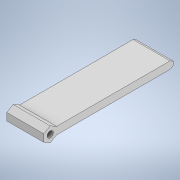
# Autodesk Inventor part: HexFlipper
Saved by Autodesk Inventor 2020 (Build 240168000, 168)
## iProperties
Created: 2023-12-22
Part Number: HexFlipper
Material: Generic
Document SubType Name: Modeling
Designer: smz3rm
Density: 1 g/cm^3
Appearance: Default
Author: smz3rm
Autodesk Inventor part; units mm, degrees
ref_plane "YZ Plane" through (0, 0, 0) normal (1, 0, 0) x (0, 1, 0)
ref_plane "XZ Plane" through (0, 0, 0) normal (0, 1, 0) x (-1, 0, 0)
ref_plane "XY Plane" through (0, 0, 0) normal (0, 0, 1) x (1, 0, 0)
sketch "Sketch1" plane through (0, 0, 0) normal (1, 0, 0) x (0, 1, 0)
  line L0 (2, 35) -> (-2, 35)
  line L1 (-2, 35) -> (-2, -35)
  line L2 (-2, -35) -> (2, -35)
  line L3 (2, -35) -> (2, 35)
  line L4 (2, 35) -> (-2, -35) construction
  line L5 (-2, 35) -> (2, -35) construction
  line L6 (-1, -35) -> (-2, -33.2679)
  line L7 (-2, -33.2679) -> (-1, -31.5359)
  line L8 (-1, -31.5359) -> (1, -31.5359)
  line L9 (1, -31.5359) -> (2, -33.2679)
  line L10 (2, -33.2679) -> (1, -35)
  line L11 (1, -35) -> (-1, -35)
  line L12 (4, 31.5359) -> (2, 28.0718)
  line L13 (2, 28.0718) -> (-2, 28.0718)
  line L14 (-2, 28.0718) -> (-4, 31.5359)
  line L15 (-4, 31.5359) -> (-2, 35)
  line L16 (-2, 35) -> (2, 35)
  line L17 (2, 35) -> (4, 31.5359)
  circle A0 centre (0, 31.5359) radius 1.65
  point P0 (0, 0)
  point P1 (0, -33.2679)
  dimension "d0" = 4
  dimension "d1" = 70
  dimension "d2" = 3.3
  constraints: 36 end point, 4 point on line, 2 midpoint, 2 parallel, 1 centre point, 1 coincident, 1 horizontal, 1 perpendicular, 26 other
  measures "d0" distance of L2.end L1.end
  measures "d1" distance of L1.end L0.end
  measures "d2" diameter of A0
extrude "Extrusion1" add sketch "Sketch1" along normal blind 20 contours L3 L13 L1 L0 | L17 L12 L3 | L1 L14 L15 | L3 L9 L8 L7 L1 L13 | L10 L2 L6 L7 L8 L9
ref_plane "Work Plane1" through (0, 2, 28.0718) normal (0, 0, -1) x (1, 0, 0)
sketch "Sketch2" plane through (0, -1, -35) normal (0, 0, -1) x (-1, 0, 0)
  line L0 (0, 2) -> (-20, 2) projected
  line L1 (0, 0) -> (-20, 0) projected
  line L2 (-10, 2) -> (-10, 0)
  circle A0 centre (-10, 1) radius 1
  point P0 (0, 1)
  dimension "d5" = 2
  constraints: 3 midpoint, 2 end point, 1 centre point, 1 vertical
  measures "d5" diameter of A0
extrude "Extrusion2" cut sketch "Sketch2" against normal up to surface (63.0718 mm away)
equation "\"d0\" = FlipperThickness"
equation "\"d1\" = FlipperLength"
equation "\"d3\" = FlipperWidth"
equation "\"d5\" = FlipperTubeDia"
equation "\"d6\" = FlipperWidth"
equation "\"FlipperThickness\" = 4"
equation "\"FlipperLength\" = 70"
equation "\"FlipperWidth\" = 20"
equation "\"FlipperTubeDia\" = 2"
body "Solid1"
